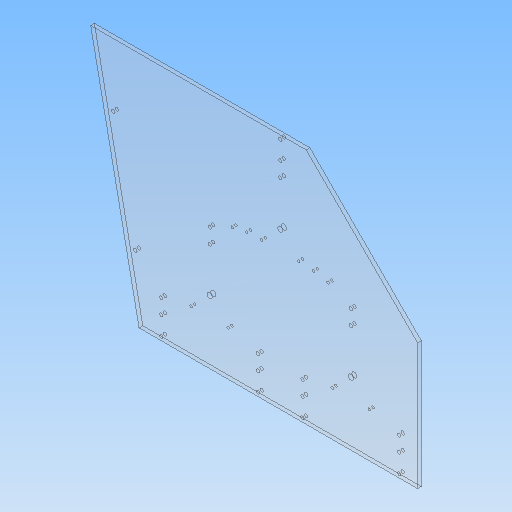
# Autodesk Inventor part: Top_Separator Backboard
Saved by Autodesk Inventor 2018.1 (Build 221171000, 171)
## iProperties
Created: 2019-03-20
Part Number: Top_Separator Backboard
Material: PMMA Plastic
Document SubType Name: Modeling
Designer: James
Density: 1.188 g/cm^3
Appearance: Polycarbonate - Clear
Mass: 704.642 g
Surface Area: 2464.7 cm^2
Volume: 593.133 cm^3
Author: James
Autodesk Inventor part; units mm, degrees
ref_plane "YZ Plane" through (0, 0, 0) normal (1, 0, 0) x (0, 1, 0)
ref_plane "XZ Plane" through (0, 0, 0) normal (0, 1, 0) x (-1, 0, 0)
ref_plane "XY Plane" through (0, 0, 0) normal (0, 0, 1) x (1, 0, 0)
sketch "Sketch1" plane through (0, 0, 0) normal (0, 0, 1) x (1, 0, 0)
  line L0 (0, 0) -> (-65.1047, 320)
  line L1 (-65.1047, 320) -> (375, 320)
  line L2 (375, 320) -> (375, 0)
  line L3 (375, 0) -> (0, 0)
  dimension "d0" = 320
  dimension "d1" = 78.5
  dimension "d2" = 375
  constraints: 8 end point, 2 perpendicular, 1 horizontal
  measures "d0" distance of L1.end L2.end
  measures "d1" angle of L3 L0
  measures "d2" distance of L2.end L0.start
extrude "Extrusion1" add sketch "Sketch1" along normal blind 5
sketch "Sketch2" plane through (0, 0, 5) normal (0, 0, 1) x (1, 0, 0)
  line L0 (0, 0) -> (375, 0) projected
  point P0 (190, 290)
  point P1 (190, 270)
  point P2 (95, 165)
  point P3 (95, 145)
  point P4 (285, 165)
  point P5 (285, 145)
  point P6 (30, 50)
  point P7 (30, 30)
  point P8 (160, 50)
  point P9 (160, 30)
  point P10 (220, 50)
  point P11 (220, 30)
  point P12 (350, 50)
  point P13 (350, 30)
  point P14 (190, 315)
  point P15 (30, 5)
  point P16 (160, 5)
  point P17 (220, 5)
  point P18 (350, 5)
  dimension "d5" = 20
  dimension "d6" = 20
  dimension "d7" = 20
  dimension "d15" = 25
  dimension "d16" = 105
  dimension "d17" = 95
  dimension "d19" = 25
  dimension "d20" = 5
  dimension "d21" = 30
  dimension "d29" = 60
  dimension "d30" = 130
  dimension "d31" = 130
  dimension "d32" = 65
  dimension "d33" = 65
  dimension "d35" = 190
  dimension "d36" = 95
  constraints: 12 vertical alignment, 11 horizontal alignment
  measures "d5" distance of point (285, 145) point (285, 165)
  measures "d6" distance of point (350, 30) point (350, 50)
  measures "d7" distance of point (190, 270) point (190, 290)
  measures "d15" distance of point (190, 315) point (190, 290)
  measures "d16" vertical distance of point (285, 165) point (190, 270)
  measures "d17" vertical distance of point (350, 50) point (285, 145)
  measures "d19" distance of point (350, 5) point (350, 30)
  measures "d20" distance from line of L0 point (30, 5)
  measures "d21" horizontal distance of point (30, 5) L0.start
  measures "d29" distance of point (220, 50) point (160, 50)
  measures "d30" distance of point (160, 5) point (30, 5)
  measures "d31" distance of point (350, 5) point (220, 5)
  measures "d32" horizontal distance of point (30, 50) point (95, 145)
  measures "d33" horizontal distance of point (220, 50) point (285, 145)
  measures "d35" distance of point (285, 165) point (95, 165)
  measures "d36" horizontal distance of point (95, 165) point (190, 270)
hole "Hole1" at (190, 290, 5) at (190, 270, 5) at (95, 165, 5) at (95, 145, 5) at (285, 165, 5) at (285, 145, 5) at (30, 50, 5) at (30, 30, 5) at (160, 50, 5) at (160, 30, 5) at (220, 50, 5) at (220, 30, 5) at (350, 50, 5) at (350, 30, 5) at (190, 315, 5) at (30, 5, 5) at (160, 5, 5) at (220, 5, 5) at (350, 5, 5) direction (0, 0, -1) diameter 4.5 end through all clearance for "Flat Head Machine Screw" size "M4" standard "Ansi Metric M Profile"
sketch "Sketch3" plane through (0, 0, 5) normal (0, 0, 1) x (1, 0, 0)
  circle A0 centre (220, 5) radius 2.25 projected
  circle A1 centre (30, 5) radius 2.25 projected
  circle A2 centre (220, 30) radius 2.25 projected
  circle A3 centre (160, 30) radius 2.25 projected
  circle A4 centre (30, 30) radius 2.25 projected
  circle A5 centre (285, 145) radius 2.25 projected
  circle A6 centre (95, 145) radius 2.25 projected
  circle A7 centre (190, 270) radius 2.25 projected
  circle A8 centre (190, 290) radius 2.25 projected
  circle A9 centre (95, 165) radius 2.25 projected
  circle A10 centre (285, 165) radius 2.25 projected
  circle A11 centre (30, 50) radius 2.25 projected
  circle A12 centre (160, 50) radius 2.25 projected
  circle A13 centre (220, 50) radius 2.25 projected
  circle A14 centre (160, 5) radius 2.25 projected
  line L0 (-65.1047, 320) -> (0, 0) projected
  line L1 (0, 0) -> (375, 0) projected
  line L2 (375, 0) -> (375, 320) projected
  line L3 (375, 320) -> (-65.1047, 320) projected
  point P0 (190, 210)
  point P1 (95, 85)
  point P2 (285, 85)
  dimension "d37" = 60
  dimension "d38" = 60
  constraints: 3 vertical alignment, 1 horizontal alignment
  measures "d37" distance of A7.centre point (190, 210)
  measures "d38" distance of A5.centre point (285, 85)
hole "Hole2" at (190, 210, 5) at (95, 85, 5) at (285, 85, 5) direction (0, 0, -1) diameter 7 end through all
sketch "Sketch4" plane through (0, 0, 5) normal (0, 0, 1) x (1, 0, 0)
  circle A0 centre (95, 85) radius 3.5 projected
  circle A1 centre (190, 210) radius 3.5 projected
  circle A2 centre (285, 85) radius 3.5 projected
  circle A3 centre (220, 5) radius 2.25 projected
  circle A4 centre (30, 5) radius 2.25 projected
  circle A5 centre (220, 30) radius 2.25 projected
  circle A6 centre (160, 30) radius 2.25 projected
  circle A7 centre (30, 30) radius 2.25 projected
  circle A8 centre (285, 145) radius 2.25 projected
  circle A9 centre (95, 145) radius 2.25 projected
  circle A10 centre (190, 270) radius 2.25 projected
  circle A11 centre (190, 290) radius 2.25 projected
  circle A12 centre (95, 165) radius 2.25 projected
  circle A13 centre (285, 165) radius 2.25 projected
  circle A14 centre (30, 50) radius 2.25 projected
  circle A15 centre (160, 50) radius 2.25 projected
  circle A16 centre (220, 50) radius 2.25 projected
  circle A17 centre (160, 5) radius 2.25 projected
  line L0 (-65.1047, 320) -> (0, 0) projected
  line L1 (0, 0) -> (375, 0) projected
  line L2 (375, 0) -> (375, 320) projected
  line L3 (375, 320) -> (-65.1047, 320) projected
  point P0 (215, 185)
  point P1 (165, 185)
  point P2 (70, 60)
  point P3 (120, 60)
  point P4 (260, 60)
  point P5 (310, 60)
  dimension "d46" = 25
  dimension "d47" = 25
  dimension "d48" = 50
  dimension "d49" = 50
  dimension "d50" = 25
  dimension "d51" = 50
  dimension "d52" = 25
  dimension "d53" = 25
  constraints: 4 horizontal alignment
  measures "d46" horizontal distance of A1.centre point (165, 185)
  measures "d47" horizontal distance of A1.centre point (165, 185)
  measures "d48" distance of point (215, 185) point (165, 185)
  measures "d49" distance of point (70, 60) point (120, 60)
  measures "d50" horizontal distance of A0.centre point (70, 60)
  measures "d51" distance of point (310, 60) point (260, 60)
  measures "d52" horizontal distance of A2.centre point (260, 60)
  measures "d53" horizontal distance of point (310, 60) A2.centre
hole "Hole3" at (215, 185, 5) at (165, 185, 5) at (70, 60, 5) at (120, 60, 5) at (260, 60, 5) at (310, 60, 5) direction (0, 0, -1) diameter 3.4 end through all clearance for "Flat Head Machine Screw" size "M3" standard "Ansi Metric M Profile"
chamfer "Chamfer1" distance 150 angle 45 1 edges at (375, 320, 2.5)
sketch "Sketch5" plane through (0, 0, 5) normal (0, 0, 1) x (1, 0, 0)
  line L0 (-65.1047, 320) -> (0, 0) projected
  line L1 (225, 320) -> (-65.1047, 320) projected
  line L2 (0, 0) -> (375, 0) projected
  point P0 (-35.0552, 235)
  point P1 (-5.15, 88.0113)
  dimension "d64" = 12.5
  dimension "d65" = 12.5
  dimension "d66" = 150
  dimension "d67" = 85
  dimension "d68" = 88.0113
  measures "d64" distance from line of point (-35.055, 235) L0
  measures "d65" distance from line of L0 point (-5.15, 88.011)
  measures "d66" distance of point (-35.055, 235) point (-5.15, 88.011)
  measures "d67" distance from line of L1 point (-35.055, 235)
  measures "d68" distance from line of L2 point (-5.15, 88.011)
hole "Hole4" at (-35.0552, 235, 5) at (-5.15, 88.0113, 5) direction (0, 0, -1) diameter 4.5 end through all clearance for "Flat Head Machine Screw" size "M4" standard "Ansi Metric M Profile"
sketch "Sketch6" plane through (0, 0, 5) normal (0, 0, 1) x (1, 0, 0)
  circle A0 centre (-35.0552, 235) radius 2.25 projected
  circle A1 centre (-5.15, 88.0113) radius 2.25 projected
  line L0 (225, 320) -> (375, 170) projected
  line L1 (225, 320) -> (-65.1047, 320) projected
  line L2 (-65.1047, 320) -> (0, 0) projected
  line L3 (0, 0) -> (375, 0) projected
  line L4 (375, 0) -> (375, 170) projected
  circle A2 centre (260, 60) radius 1.7 projected
  circle A3 centre (70, 60) radius 1.7 projected
  circle A4 centre (215, 185) radius 1.7 projected
  circle A5 centre (165, 185) radius 1.7 projected
  circle A6 centre (120, 60) radius 1.7 projected
  circle A7 centre (310, 60) radius 1.7 projected
  circle A8 centre (95, 85) radius 3.5 projected
  circle A9 centre (190, 210) radius 3.5 projected
  circle A10 centre (285, 85) radius 3.5 projected
  circle A11 centre (220, 5) radius 2.25 projected
  circle A12 centre (30, 5) radius 2.25 projected
  circle A13 centre (350, 30) radius 2.25 projected
  circle A14 centre (220, 30) radius 2.25 projected
  circle A15 centre (160, 30) radius 2.25 projected
  circle A16 centre (30, 30) radius 2.25 projected
  circle A17 centre (285, 145) radius 2.25 projected
  circle A18 centre (95, 145) radius 2.25 projected
  circle A19 centre (190, 270) radius 2.25 projected
  circle A20 centre (190, 290) radius 2.25 projected
  circle A21 centre (95, 165) radius 2.25 projected
  circle A22 centre (285, 165) radius 2.25 projected
  circle A23 centre (30, 50) radius 2.25 projected
  circle A24 centre (160, 50) radius 2.25 projected
  circle A25 centre (220, 50) radius 2.25 projected
  circle A26 centre (350, 50) radius 2.25 projected
  circle A27 centre (190, 315) radius 2.25 projected
  circle A28 centre (160, 5) radius 2.25 projected
  circle A29 centre (350, 5) radius 2.25 projected
  point P0 (125.4041, 180)
  point P1 (145, 184)
  point P2 (235, 184)
  point P3 (254.5959, 180)
  dimension "d76" = 20
  dimension "d77" = 4
  dimension "d78" = 20
  dimension "d79" = 45
  dimension "d80" = 26
  dimension "d81" = 45
  constraints: 2 horizontal alignment
  measures "d76" distance of point (145, 184) point (125.404, 180)
  measures "d77" vertical distance of point (125.404, 180) point (145, 184)
  measures "d78" distance of point (254.596, 180) point (235, 184)
  measures "d79" horizontal distance of A9.centre point (145, 184)
  measures "d80" vertical distance of A9.centre point (145, 184)
  measures "d81" horizontal distance of point (235, 184) A9.centre
hole "Hole5" at (125.4041, 180, 5) at (145, 184, 5) at (235, 184, 5) at (254.5959, 180, 5) direction (0, 0, -1) diameter 3.4 end through all clearance for "Flat Head Machine Screw" size "M3" standard "Ansi Metric M Profile"
equation "\"d5\" = d6"
equation "\"d7\" = d5"
equation "\"d31\" = d30"
equation "\"d32\" = 0.5 * d30"
equation "\"d33\" = 0.5 * d31"
equation "\"d36\" = 0.5 * d35"
equation "\"d38\" = d37"
equation "\"d48\" = 2 * d47"
equation "\"d49\" = d48"
equation "\"d50\" = 0.5 * d49"
equation "\"d51\" = d49"
equation "\"d52\" = 0.5 * d51"
equation "\"d53\" = d46"
equation "\"d65\" = d64"
equation "\"d78\" = d76"
equation "\"d81\" = d79"
body "Solid1"
